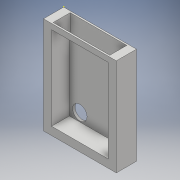
# Autodesk Inventor part: Case_Top_Part
Saved by Autodesk Inventor 2017 (Build 210142000, 142)
## iProperties
Created: 2020-01-23
Part Number: Case_Top_Part
Material: Generic
Document SubType Name: Modeling
Designer: Manny
Density: 1 g/cm^3
Appearance: Default
Author: Manny
Autodesk Inventor part; units mm, degrees
ref_plane "YZ Plane" through (0, 0, 0) normal (1, 0, 0) x (0, 1, 0)
ref_plane "XZ Plane" through (0, 0, 0) normal (0, 1, 0) x (-1, 0, 0)
ref_plane "XY Plane" through (0, 0, 0) normal (0, 0, 1) x (1, 0, 0)
sketch "Sketch1" plane through (0, 0, 0) normal (0, 1, 0) x (-1, 0, 0)
  line L0 (0, 0) -> (-90, 0)
  line L1 (-90, 0) -> (-90, -120)
  line L2 (-90, -120) -> (0, -120)
  line L3 (0, -120) -> (0, 0)
  dimension "d0" = 90
  dimension "d1" = 120
  constraints: 8 end point, 2 parallel, 1 horizontal, 1 perpendicular
  measures "d0" distance of L1.end L2.end
  measures "d1" distance of L0.end L1.end
extrude "Extrusion1" add sketch "Sketch1" along normal blind 25
sketch "Sketch2" plane through (0, 0, 0) normal (0, -1, 0) x (1, 0, 0)
  line L0 (80, -6.6572) -> (10, -6.6572)
  line L1 (10, -6.6572) -> (10, -110)
  line L2 (10, -110) -> (80, -110)
  line L3 (80, -110) -> (80, -6.6572)
  line L4 (0, -120) -> (0, 0) projected
  line L5 (0, 0) -> (90, 0) projected
  line L6 (90, -120) -> (0, -120) projected
  line L7 (90, 0) -> (90, -120) projected
  dimension "d4" = 10
  dimension "d5" = 6.6572
  dimension "d6" = 10
  dimension "d7" = 10
  constraints: 8 end point, 2 parallel, 1 horizontal, 1 perpendicular
  measures "d4" distance between parallel lines of L4 L1
  measures "d5" distance between parallel lines of L5 L0
  measures "d6" distance between parallel lines of L6 L2
  measures "d7" distance between parallel lines of L7 L3
extrude "Extrusion2" cut sketch "Sketch2" against normal blind 22 contours L3 L2 L1 L0
sketch "Sketch3" plane through (0, 25, 0) normal (0, 1, 0) x (1, 0, 0)
  point P0 (0, 0)
sketch "Sketch4" plane through (0, 22, 0) normal (0, -1, 0) x (1, 0, 0)
  circle A0 centre (22.9438, -100) radius 8.9417
  line L0 (90, -120) -> (0, -120) projected
  point P0 (0, 0)
  dimension "d10" = 20
  dimension "d19" = 17.8834
  constraints: 1 centre point
  measures "d10" distance from line of L0 A0.centre
  measures "d19" diameter of A0
extrude "Extrusion3" cut sketch "Sketch4" against normal blind 22
sketch "Sketch5" plane through (0, 0, 0) normal (0, 0, 1) x (1, 0, 0)
  line L0 (10, 23) -> (80, 23)
  line L1 (80, 23) -> (80, 2)
  line L2 (80, 2) -> (10, 2)
  line L3 (10, 2) -> (10, 23)
  line L4 (0, 0) -> (0, 25) projected
  line L5 (90, 0) -> (90, 25) projected
  line L6 (0, 0) -> (90, 0) projected
  line L7 (90, 25) -> (0, 25) projected
  dimension "d13" = 10
  dimension "d14" = 10
  dimension "d15" = 2
  dimension "d16" = 2
  constraints: 8 end point, 2 parallel, 1 horizontal, 1 perpendicular
  measures "d13" distance between parallel lines of L4 L3
  measures "d14" distance between parallel lines of L5 L1
  measures "d15" distance between parallel lines of L6 L2
  measures "d16" distance between parallel lines of L7 L0
extrude "Extrusion4" cut sketch "Sketch5" against normal blind 22 contours L0 L1 L2 L3
body "Solid1"
